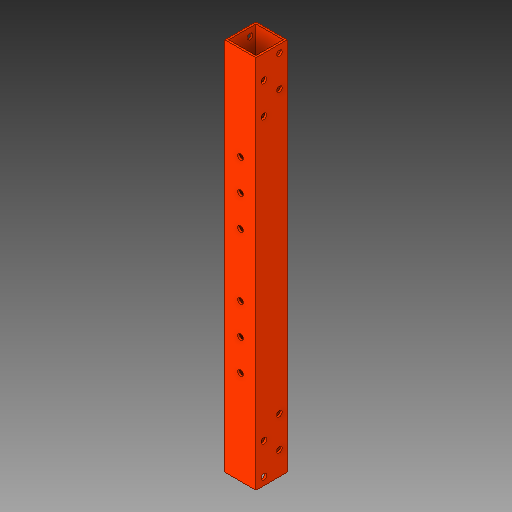
# Autodesk Inventor part: ElvCrossBeam
Saved by Autodesk Inventor 2019 (Build 230136000, 136)
## iProperties
Created: 2019-01-09
Part Number: ElvCrossBeam
Material: Aluminum 6061
Document SubType Name: Modeling
Designer: james
Density: 2.7 g/cm^3
Appearance: Default(1)
Mass: 122.277 g
Surface Area: 580.266 cm^2
Volume: 45.2877 cm^3
Author: james
Autodesk Inventor part; units mm, degrees
ref_plane "YZ Plane" through (0, 0, 0) normal (1, 0, 0) x (0, 1, 0)
ref_plane "XZ Plane" through (0, 0, 0) normal (0, 1, 0) x (-1, 0, 0)
ref_plane "XY Plane" through (0, 0, 0) normal (0, 0, 1) x (1, 0, 0)
sketch "Sketch1" plane through (0, 0, 0) normal (0, 1, 0) x (-1, 0, 0)
  line L0 (17.0295, 14.999) -> (-8.3705, 14.999)
  line L1 (-8.3705, 14.999) -> (-8.3705, -10.401)
  line L2 (-8.3705, -10.401) -> (17.0295, -10.401)
  line L3 (17.0295, -10.401) -> (17.0295, 14.999)
  line L4 (15.442, -8.8135) -> (-6.783, -8.8135)
  line L5 (-6.783, -8.8135) -> (-6.783, 13.4115)
  line L6 (-6.783, 13.4115) -> (15.442, 13.4115)
  line L7 (15.442, 13.4115) -> (15.442, -8.8135)
  point P0 (0, 0)
  dimension "d0" = 25.4
  dimension "d1" = 25.4
  dimension "d4" = 1.5875
  dimension "d5" = 1.5875
  dimension "d6" = 1.5875
  dimension "d7" = 1.5875
  constraints: 16 end point, 4 parallel, 2 horizontal, 2 perpendicular
  measures "d0" distance of L0.end L1.end
  measures "d1" distance of L0.start L0.end
  measures "d4" distance between parallel lines of L0 L6
  measures "d5" distance between parallel lines of L2 L4
  measures "d6" distance between parallel lines of L3 L7
  measures "d7" distance between parallel lines of L1 L5
extrude "Extrusion2" add sketch "Sketch1" along normal blind 304.8
sketch "Sketch2" plane through (8.3705, 0, 14.999) normal (1, 0, 0) x (0, 0, -1)
  line L0 (0, 304.8) -> (25.4, 304.8) projected
  line L1 (25.4, 0) -> (25.4, 304.8) projected
  line L2 (0, 0) -> (0, 304.8) projected
  point P0 (14.999, 0)
  point P1 (19.05, 298.45)
  point P2 (19.05, 273.05)
  point P3 (6.35, 285.75)
  point P4 (6.35, 260.35)
  dimension "d10" = 6.35
  dimension "d11" = 6.35
  dimension "d12" = 6.35
  dimension "d13" = 25.4
  dimension "d14" = 6.35
  dimension "d15" = 25.4
  dimension "d16" = 6.35
  dimension "d17" = 19.05
  measures "d10" distance from line of L0 point (19.05, 298.45)
  measures "d11" distance from line of L1 point (19.05, 298.45)
  measures "d12" distance from line of L1 point (19.05, 273.05)
  measures "d13" distance of point (19.05, 298.45) point (19.05, 273.05)
  measures "d14" distance from line of L2 point (6.35, 285.75)
  measures "d15" distance of point (6.35, 260.35) point (6.35, 285.75)
  measures "d16" distance from line of L2 point (6.35, 260.35)
  measures "d17" distance from line of L0 point (6.35, 285.75)
hole "Hole1" at (8.3705, 298.45, -4.051) at (8.3705, 273.05, -4.051) at (8.3705, 285.75, 8.649) at (8.3705, 260.35, 8.649) direction (-1, 0, 0) diameter 4.7625 depth 25.4 tip angle 118
sketch "Sketch3" plane through (8.3705, 0, 14.999) normal (1, 0, 0) x (0, 0, -1)
  line L0 (25.4, 0) -> (25.4, 304.8) projected
  line L1 (0, 0) -> (25.4, 0) projected
  line L2 (0, 0) -> (0, 304.8) projected
  point P0 (14.999, 0)
  point P1 (6.35, 6.35)
  point P2 (19.05, 19.05)
  point P3 (6.35, 31.75)
  point P4 (19.05, 44.45)
  dimension "d25" = 6.35
  dimension "d26" = 6.35
  dimension "d27" = 19.05
  dimension "d28" = 25.4
  dimension "d29" = 6.35
  dimension "d30" = 6.35
  dimension "d31" = 6.35
  dimension "d32" = 25.4
  measures "d25" distance from line of L0 point (19.05, 44.45)
  measures "d26" distance from line of L0 point (19.05, 19.05)
  measures "d27" distance from line of L1 point (19.05, 19.05)
  measures "d28" distance of point (19.05, 44.45) point (19.05, 19.05)
  measures "d29" distance from line of L1 point (6.35, 6.35)
  measures "d30" distance from line of L2 point (6.35, 6.35)
  measures "d31" distance from line of L2 point (6.35, 31.75)
  measures "d32" distance of point (6.35, 6.35) point (6.35, 31.75)
hole "Hole2" at (8.3705, 6.35, 8.649) at (8.3705, 19.05, -4.051) at (8.3705, 31.75, 8.649) at (8.3705, 44.45, -4.051) direction (-1, 0, 0) diameter 4.7625 depth 25.4 tip angle 118
sketch "Sketch4" plane through (-17.0295, 0, 14.999) normal (0, 0, 1) x (1, 0, 0)
  line L0 (0, 0) -> (0, 304.8) projected
  line L1 (0, 0) -> (25.4, 0) projected
  line L2 (0, 304.8) -> (25.4, 304.8) projected
  point P0 (17.0295, 0)
  point P1 (12.7, 76.2)
  point P2 (12.7, 101.6)
  point P3 (12.7, 127)
  point P4 (12.7, 177.8)
  point P5 (12.7, 228.6)
  point P6 (12.7, 203.2)
  dimension "d40" = 12.7
  dimension "d41" = 12.7
  dimension "d42" = 12.7
  dimension "d43" = 25.4
  dimension "d44" = 25.4
  dimension "d45" = 76.2
  dimension "d46" = 12.7
  dimension "d47" = 12.7
  dimension "d48" = 12.7
  dimension "d49" = 25.4
  dimension "d50" = 25.4
  dimension "d51" = 76.2
  measures "d40" distance from line of L0 point (12.7, 127)
  measures "d41" distance from line of L0 point (12.7, 101.6)
  measures "d42" distance from line of L0 point (12.7, 76.2)
  measures "d43" distance of point (12.7, 101.6) point (12.7, 76.2)
  measures "d44" distance of point (12.7, 101.6) point (12.7, 127)
  measures "d45" distance from line of L1 point (12.7, 76.2)
  measures "d46" distance from line of L0 point (12.7, 177.8)
  measures "d47" distance from line of L0 point (12.7, 228.6)
  measures "d48" distance from line of L0 point (12.7, 203.2)
  measures "d49" distance of point (12.7, 228.6) point (12.7, 203.2)
  measures "d50" distance of point (12.7, 177.8) point (12.7, 203.2)
  measures "d51" distance from line of L2 point (12.7, 228.6)
hole "Hole3" at (-4.3295, 76.2, 14.999) at (-4.3295, 101.6, 14.999) at (-4.3295, 127, 14.999) at (-4.3295, 177.8, 14.999) at (-4.3295, 228.6, 14.999) at (-4.3295, 203.2, 14.999) direction (0, 0, -1) diameter 4.826 depth 25.4 tip angle 118.188
equation "\"d0\" = ElvBeamWidth"
equation "\"d1\" = ElvBeamWidth"
equation "\"d4\" = ElvWallWidth"
equation "\"d5\" = ElvWallWidth"
equation "\"d6\" = ElvWallWidth"
equation "\"d7\" = ElvWallWidth"
equation "\"d8\" = ElvCrossBeamLength"
equation "\"ElvMiddleBeamLength\" = 990.6"
equation "\"ElvWallWidth\" = 1.5875"
equation "\"ElvFrontBeamLength\" = 990.6"
equation "\"ElvEndEffectLength\" = 419.1"
equation "\"ElvCrossBeamLength\" = 304.8"
equation "\"ElvBeamWidth\" = 25.4"
equation "\"ElvFrontBeamLength_1\" = 1066.8"
equation "\"ElvFixedBeamLength\" = 990.6"
equation "\"ElvDelHeight\" = 101.6"
equation "\"ElvDelFrontTabLength\" = 6.35"
equation "\"ElvDelWidth\" = 18.542"
equation "\"ElvDelDepth\" = 6.35"
equation "\"ElvTopBeamLength\" = 457.2"
equation "\"ElvHoleFromBottom\" = 38.1"
equation "\"ElvHoleFromMid\" = 38.1"
equation "\"ElvHoleFromFixed\" = 50.8"
equation "\"ElvHoleFromFront\" = 25.4"
equation "\"ElvRivetPlateLength\" = 76.2"
equation "\"ElvDelMiddleTabLength\" = 6.35"
body "Solid2"
